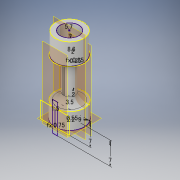
# Autodesk Inventor part: モータジョイント
Saved by Autodesk Inventor 2019.3 (Build 233278000, 278)
## iProperties
Created: 2019-08-08
Part Number: モータジョイント
Material: Generic
Document SubType Name: Modeling
Designer: ushiyama
Density: 1 g/cm^3
Appearance: Default
Author: ushiyama
Autodesk Inventor part; units mm, degrees
ref_plane "YZ Plane" through (0, 0, 0) normal (1, 0, 0) x (0, 1, 0)
sketch "スケッチ2" plane through (0, 0, 0) normal (0, 1, 0) x (-1, 0, 0)
  circle A0 centre (0, 0) radius 4.5
  dimension "d9" = 9
  constraints: 1 centre point, 1 coincident
  measures "d9" diameter of A0
sketch "スケッチ1" plane through (0, 0, 0) normal (0, 1, 0) x (-1, 0, 0)
  arc A0 (-0.55, -0.9526) -> (-0.55, 0.9526) centre (0, 0) ccw
  line L0 (-0.55, -0.9526) -> (-0.55, 0.9526)
  dimension "d0" = 2.2
  dimension "d2" = 0.55
  constraints: 2 end point, 2 point on circle, 1 centre point, 1 coincident, 1 vertical
  measures "d0" diameter of A0
  measures "d2" distance from line of point (0, 0) L0
extrude "押し出し1" add sketch "スケッチ2" along normal blind 5
extrude "押し出し2" cut sketch "スケッチ1" along normal blind 3
ref_plane "作業平面2" through (0, 0, 4.5) normal (0, 0, 1) x (1, 0, 0)
sketch "スケッチ4" plane through (0, 0, 4.5) normal (0, 0, 1) x (1, 0, 0)
  line L0 (4.5, 5) -> (-4.5, 5) projected
  line L1 (-4.5, 0) -> (4.5, 0) projected
  line L2 (4.5, 0) -> (4.5, 5) projected
  line L3 (-4.5, 0) -> (-4.5, 5) projected
  line L4 (-0.75, 7) -> (0.75, 7)
  line L5 (0.75, 7) -> (0.75, -2)
  line L6 (0.75, -2) -> (-0.75, -2)
  line L7 (-0.75, -2) -> (-0.75, 7)
  line L8 (0, 5) -> (0, 0)
  dimension "d14" = 7
  dimension "d15" = 7
  dimension "d16" = 1.5
  dimension "d18" = 0.75
  constraints: 10 end point, 2 parallel, 1 horizontal, 1 midpoint, 1 perpendicular, 1 vertical
  measures "d14" distance between parallel lines of L1 L4
  measures "d15" distance between parallel lines of L0 L6
  measures "d16" distance between parallel lines of L5 L7
  measures "d18" distance between parallel lines of L5 L8
sketch "スケッチ3" plane through (0, 5, 0) normal (0, 1, 0) x (1, 0, 0)
  circle A0 centre (0, 0) radius 4.5 projected
  circle A1 centre (0, 0) radius 1.75
  dimension "d11" = 3.5
  constraints: 1 centre point, 1 coincident
  measures "d11" diameter of A1
extrude "押し出し6" add sketch "スケッチ3" along normal blind 12 contours A1
ref_plane "作業平面3" through (0, 17, 0) normal (0, 1, 0) x (1, 0, 0)
sketch "スケッチ5" plane through (0, 17, 0) normal (0, 1, 0) x (1, 0, 0)
  circle A0 centre (0, 0) radius 4.5 projected
  circle A1 centre (0, 0) radius 4.3
  dimension "d29" = 8.6
  constraints: 1 centre point, 1 coincident
  measures "d29" diameter of A1
extrude "押し出し8" add sketch "スケッチ5" along normal blind 6.5 contours A1
sketch "スケッチ7" plane through (0, 23.5, 0) normal (0, 1, 0) x (1, 0, 0)
  circle A0 centre (0, 0) radius 2.85
  circle A1 centre (0, 0) radius 4.3 projected
  dimension "d32" = 5.7
  constraints: 1 centre point, 1 coincident
  measures "d32" diameter of A0
extrude "押し出し9" cut sketch "スケッチ7" against normal blind 4 contours A0
ref_plane "作業平面4" through (0, 5, -1.75) normal (0, 0, 1) x (1, 0, 0)
sketch "スケッチ8" plane through (0, 5, -1.75) normal (0, 0, 1) x (1, 0, 0)
  line L0 (0.25, 10) -> (-0.25, 10)
  line L1 (-0.25, 10) -> (-0.25, 2)
  line L2 (-0.25, 2) -> (0.25, 2)
  line L3 (0.25, 2) -> (0.25, 10)
  line L4 (0, 7.5314) -> (0, 7.4819)
  line L5 (-4.3, 12) -> (4.3, 12) projected
  line L6 (4.5, 0) -> (-4.5, 0) projected
  line L7 (0, 12) -> (0, 0)
  point P0 (0, -5)
  point P1 (0, 10)
  point P2 (0, 10)
  dimension "d36" = 0.25
  dimension "d37" = 0.25
  dimension "d40" = 2
  dimension "d41" = 2
  constraints: 12 end point, 4 midpoint, 2 parallel, 2 vertical, 1 horizontal, 1 perpendicular, 1 point on line
  measures "d36" distance from line of L3 point (0, 10)
  measures "d37" distance from line of point (0, 10) L1
  measures "d40" distance between parallel lines of L5 L0
  measures "d41" distance between parallel lines of L6 L2
extrude "押し出し10" cut sketch "スケッチ8" along normal blind 5
fillet "フィレット3" radius 2 2 edges at (-1.75, 5, 0) (-1.75, 17, 0)
equation "\"d18\" = 0.5 * d16"
equation "\"d37\" = d36"
